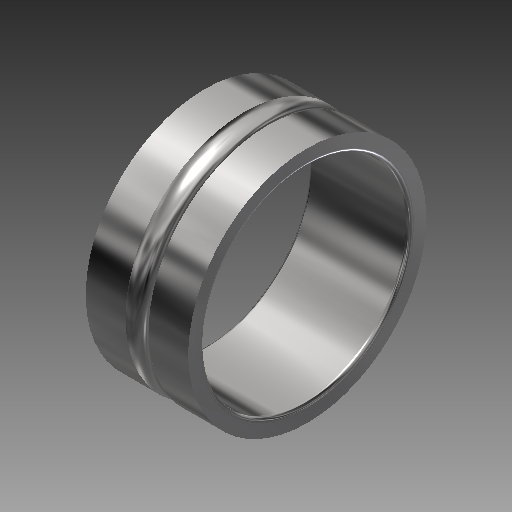
# Autodesk Inventor part: MF85ZZ Inner Ring
Saved by Autodesk Inventor 2018 (Build 220112000, 112)
## iProperties
Category: PARTsolutions
Company: NSK_RB
Created: 2016-04-26
Part Number: MF85ZZ Inner Ring
Catalog Web Link: www.cadenas.de
Description: shielded_type_zz_zzs_IR-
Vendor: NSK_RB
Document SubType Name: Modeling
Designer: psAdmin
Manufacturer: NSK_RB
Mass: 0.125568 g
Surface Area: 0.976395 cm^2
Volume: 0.0162023 cm^3
Density: 7.75 g/cm^3
Material: ステンレス鋼 440C
Appearance: 半つや出し
PSOL_IDENT_0: {$CADENAS_DATA\23d-libs\nsk_rb\roller_bearings\deep_groove_bb\exstra_small_miniatur_bb\metric_design
PSOL_IDENT_1: _with_flange\shielded_type_zz_zzs_ir_1.prj},194 {VTYP=3D},{NB=MF85ZZ Inner Ring},{LINA=MF85ZZ Inner
PSOL_IDENT_2: Ring},{NN=shielded_type_zz_zzs_IR},{DATE=18.06.2013 02:54:38},{GEOMDATE=04.01.2008 00:00:00},{VERSIO
PSOL_IDENT_3: N=},{LINEID=210},{LINESUBID=-1},{WBVAR=}  {NB=MF85ZZ Inner Ring},{LINA=MF85ZZ Inner Ring},{KT=DUMMY}
PSOL_IDENT_4: ,{IDNR=},{STAN=},{ORDER=MF85ZZ},{SD=5.0},{X=5.0},{D=8},{DD=8},{DD1=0.0},{D2=9.2},{DD2=9.2},{B=0.0},{
PSOL_IDENT_5: B1=2.5},{CC1=0.0},{C2=0.6},{CC2=0.6},{R=0.00},{R1=0.10},{DI1=5.80},{DI2=5.80},{SDE1=7.00},{SDE2=7.40
PSOL_IDENT_6: },{CR1=310},{COR1=120},{CR2=31},{COR2=12.0},{LG=53000},{LO=63000},{DA=0.0},{DB=5.8},{RA=0.00},{RB=0.
PSOL_IDENT_7: 10},{MASS=0.41},{SC=1},{N=17}
NN: shielded_type_zz_zzs_IR
NB: MF85ZZ Inner Ring
NBSYN: $ORDER. Inner Ring
LINA: MF85ZZ Inner Ring
ORDER: MF85ZZ
SD: 5.0
X: 5.0
D: 8
DD: 8
DD1: 0.0
D2: 9.2
DD2: 9.2
B: 0.0
B1: 2.5
CC1: 0.0
C2: 0.6
CC2: 0.6
R: 0.00
R1: 0.10
DI1: 5.80
DI2: 5.80
SDE1: 7.00
SDE2: 7.40
CR1: 310
COR1: 120
CR2: 31
COR2: 12.0
LG: 53000
LO: 63000
DA: 0.0
DB: 5.8
RA: 0.00
RB: 0.10
MASS: 0.41
SC: 1
SUPPLIER: NSK_RB
ARTICLENO: MF85ZZ Inner Ring
BOMINFO: MF85ZZ Inner Ring
CREATOR: CADENAS GmbH
Title: MF85ZZ Inner Ring
Author: Cadenas PARTsolutions
Autodesk Inventor part; units mm, degrees
sketch "Sketch_1" plane through (0, 0, 0) normal (0, 0, 1) x (1, 0, 0)
  line L0 (2.5, 0) -> (0, 0)
  arc A0 (0, 2.6) -> (0.1, 2.5) centre (0.1, 2.6) ccw
  line L1 (0.1, 2.5) -> (2.4, 2.5)
  arc A1 (2.4, 2.5) -> (2.5, 2.6) centre (2.4, 2.6) ccw
  line L2 (2.5, 2.6) -> (2.5, 2.9)
  line L3 (2.5, 2.9) -> (1.5328, 2.9)
  arc A2 (0.9672, 2.9) -> (1.5328, 2.9) centre (1.25, 3.25) ccw
  line L4 (0.9672, 2.9) -> (0, 2.9)
  line L5 (0, 2.9) -> (0, 2.6)
  constraints: 12 end point, 6 point on circle, 3 centre point
revolve "Revolution1" add sketch "Sketch_1" angle 360 about axis through (2.5, 0, 0) along (1, 0, 0)
ref_plane "ip_st_1_1_XY" through (1.25, 3.25, 0) normal (1, 0, 0) x (0, 0, -1)
ref_plane "ip_st_1_1_YZ" through (1.25, 3.25, 0) normal (0, 0, -1) x (0, 1, 0)
ref_plane "ip_st_1_1_ZX" through (1.25, 3.25, 0) normal (0, 1, 0) x (1, 0, 0)
ref_plane "ip_st_1_10_XY" through (1.25, -3.1947, -0.5972) normal (1, 0, 0) x (0, 0, -1)
ref_plane "ip_st_1_10_YZ" through (1.25, -3.1947, -0.5972) normal (0, 0, -1) x (0, 1, 0)
ref_plane "ip_st_1_10_ZX" through (1.25, -3.1947, -0.5972) normal (0, 1, 0) x (1, 0, 0)
ref_plane "ip_st_1_11_XY" through (1.25, -2.7632, -1.7109) normal (1, 0, 0) x (0, 0, -1)
ref_plane "ip_st_1_11_YZ" through (1.25, -2.7632, -1.7109) normal (0, 0, -1) x (0, 1, 0)
ref_plane "ip_st_1_11_ZX" through (1.25, -2.7632, -1.7109) normal (0, 1, 0) x (1, 0, 0)
ref_plane "ip_st_1_12_XY" through (1.25, -1.9586, -2.5936) normal (1, 0, 0) x (0, 0, -1)
ref_plane "ip_st_1_12_YZ" through (1.25, -1.9586, -2.5936) normal (0, 0, -1) x (0, 1, 0)
ref_plane "ip_st_1_12_ZX" through (1.25, -1.9586, -2.5936) normal (0, 1, 0) x (1, 0, 0)
ref_plane "ip_st_1_13_XY" through (1.25, -0.8894, -3.1259) normal (1, 0, 0) x (0, 0, -1)
ref_plane "ip_st_1_13_YZ" through (1.25, -0.8894, -3.1259) normal (0, 0, -1) x (0, 1, 0)
ref_plane "ip_st_1_13_ZX" through (1.25, -0.8894, -3.1259) normal (0, 1, 0) x (1, 0, 0)
ref_plane "ip_st_1_14_XY" through (1.25, 0.2999, -3.2361) normal (1, 0, 0) x (0, 0, -1)
ref_plane "ip_st_1_14_YZ" through (1.25, 0.2999, -3.2361) normal (0, 0, -1) x (0, 1, 0)
ref_plane "ip_st_1_14_ZX" through (1.25, 0.2999, -3.2361) normal (0, 1, 0) x (1, 0, 0)
ref_plane "ip_st_1_15_XY" through (1.25, 1.4486, -2.9093) normal (1, 0, 0) x (0, 0, -1)
ref_plane "ip_st_1_15_YZ" through (1.25, 1.4486, -2.9093) normal (0, 0, -1) x (0, 1, 0)
ref_plane "ip_st_1_15_ZX" through (1.25, 1.4486, -2.9093) normal (0, 1, 0) x (1, 0, 0)
ref_plane "ip_st_1_16_XY" through (1.25, 2.4018, -2.1895) normal (1, 0, 0) x (0, 0, -1)
ref_plane "ip_st_1_16_YZ" through (1.25, 2.4018, -2.1895) normal (0, 0, -1) x (0, 1, 0)
ref_plane "ip_st_1_16_ZX" through (1.25, 2.4018, -2.1895) normal (0, 1, 0) x (1, 0, 0)
ref_plane "ip_st_1_17_XY" through (1.25, 3.0305, -1.174) normal (1, 0, 0) x (0, 0, -1)
ref_plane "ip_st_1_17_YZ" through (1.25, 3.0305, -1.174) normal (0, 0, -1) x (0, 1, 0)
ref_plane "ip_st_1_17_ZX" through (1.25, 3.0305, -1.174) normal (0, 1, 0) x (1, 0, 0)
ref_plane "ip_st_1_2_XY" through (1.25, 3.0305, 1.174) normal (1, 0, 0) x (0, 0, -1)
ref_plane "ip_st_1_2_YZ" through (1.25, 3.0305, 1.174) normal (0, 0, -1) x (0, 1, 0)
ref_plane "ip_st_1_2_ZX" through (1.25, 3.0305, 1.174) normal (0, 1, 0) x (1, 0, 0)
ref_plane "ip_st_1_3_XY" through (1.25, 2.4018, 2.1895) normal (1, 0, 0) x (0, 0, -1)
ref_plane "ip_st_1_3_YZ" through (1.25, 2.4018, 2.1895) normal (0, 0, -1) x (0, 1, 0)
ref_plane "ip_st_1_3_ZX" through (1.25, 2.4018, 2.1895) normal (0, 1, 0) x (1, 0, 0)
ref_plane "ip_st_1_4_XY" through (1.25, 1.4486, 2.9093) normal (1, 0, 0) x (0, 0, -1)
ref_plane "ip_st_1_4_YZ" through (1.25, 1.4486, 2.9093) normal (0, 0, -1) x (0, 1, 0)
ref_plane "ip_st_1_4_ZX" through (1.25, 1.4486, 2.9093) normal (0, 1, 0) x (1, 0, 0)
ref_plane "ip_st_1_5_XY" through (1.25, 0.2999, 3.2361) normal (1, 0, 0) x (0, 0, -1)
ref_plane "ip_st_1_5_YZ" through (1.25, 0.2999, 3.2361) normal (0, 0, -1) x (0, 1, 0)
ref_plane "ip_st_1_5_ZX" through (1.25, 0.2999, 3.2361) normal (0, 1, 0) x (1, 0, 0)
ref_plane "ip_st_1_6_XY" through (1.25, -0.8894, 3.1259) normal (1, 0, 0) x (0, 0, -1)
ref_plane "ip_st_1_6_YZ" through (1.25, -0.8894, 3.1259) normal (0, 0, -1) x (0, 1, 0)
ref_plane "ip_st_1_6_ZX" through (1.25, -0.8894, 3.1259) normal (0, 1, 0) x (1, 0, 0)
ref_plane "ip_st_1_7_XY" through (1.25, -1.9586, 2.5936) normal (1, 0, 0) x (0, 0, -1)
ref_plane "ip_st_1_7_YZ" through (1.25, -1.9586, 2.5936) normal (0, 0, -1) x (0, 1, 0)
ref_plane "ip_st_1_7_ZX" through (1.25, -1.9586, 2.5936) normal (0, 1, 0) x (1, 0, 0)
ref_plane "ip_st_1_8_XY" through (1.25, -2.7632, 1.7109) normal (1, 0, 0) x (0, 0, -1)
ref_plane "ip_st_1_8_YZ" through (1.25, -2.7632, 1.7109) normal (0, 0, -1) x (0, 1, 0)
ref_plane "ip_st_1_8_ZX" through (1.25, -2.7632, 1.7109) normal (0, 1, 0) x (1, 0, 0)
ref_plane "ip_st_1_9_XY" through (1.25, -3.1947, 0.5972) normal (1, 0, 0) x (0, 0, -1)
ref_plane "ip_st_1_9_YZ" through (1.25, -3.1947, 0.5972) normal (0, 0, -1) x (0, 1, 0)
ref_plane "ip_st_1_9_ZX" through (1.25, -3.1947, 0.5972) normal (0, 1, 0) x (1, 0, 0)
ref_plane "ip_st_1a_XY" through (0, 0, 0) normal (1, 0, 0) x (0, 0, -1)
ref_plane "ip_st_1a_YZ" through (0, 0, 0) normal (0, 0, -1) x (0, 1, 0)
ref_plane "ip_st_1a_ZX" through (0, 0, 0) normal (0, 1, 0) x (1, 0, 0)
ref_plane "ip_st_2a_XY" through (0.1562, 0, 0) normal (1, 0, 0) x (0, 0, -1)
ref_plane "ip_st_2a_YZ" through (0.1562, 0, 0) normal (0, 0, -1) x (0, 1, 0)
ref_plane "ip_st_2a_ZX" through (0.1562, 0, 0) normal (0, 1, 0) x (1, 0, 0)
body "Solid1"
